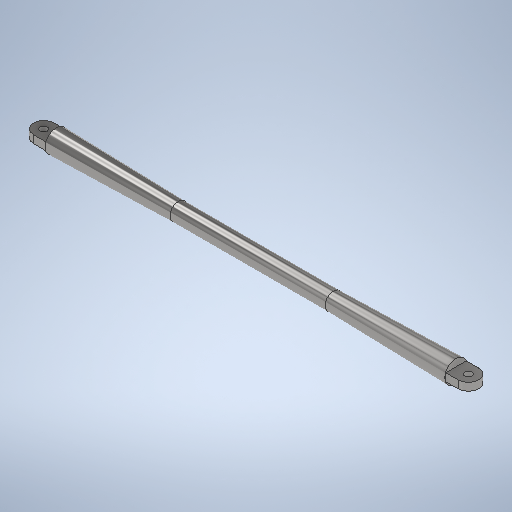
# Autodesk Inventor part: Arjun_SteeringRod
Saved by Autodesk Inventor 2025 (Build 290162000, 162)
## iProperties
Created: 2024-11-03
Part Number: Arjun_SteeringRod
Material: Generic
Document SubType Name: Modeling
Designer: pathl
Density: 1 g/cm^3
Appearance: Default
Author: pathl
Autodesk Inventor part; units mm, degrees
ref_plane "YZ Plane" through (0, 0, 0) normal (1, 0, 0) x (0, 1, 0)
ref_plane "XZ Plane" through (0, 0, 0) normal (0, 1, 0) x (-1, 0, 0)
sketch "Sketch1" plane through (0, 0, 0) normal (0, 0, 1) x (1, 0, 0)
  line L0 (0, 0) -> (575, 0)
  line L1 (575, 0) -> (575, 30)
  line L2 (575, 30) -> (200, 22)
  line L3 (200, 22) -> (0, 22)
  line L4 (0, 22) -> (0, 0)
  dimension "d0" = 575
  dimension "d1" = 30
  dimension "d2" = 22
  dimension "d3" = 200
  constraints: 10 end point, 2 perpendicular, 1 horizontal, 1 parallel
  measures "d0" distance of L0.start L0.end
  measures "d1" distance of L0.end L1.end
  measures "d2" distance of L3.end L0.start
  measures "d3" distance of L2.end L3.end
revolve "Revolution1" add sketch "Sketch1" angle 360 about axis through (0, 0, 0) along (1, 0, 0)
ref_plane "Work Plane1" through (0, 0, 30) normal (0, 0, 1) x (1, 0, 0)
sketch "Sketch2" plane through (0, 0, 30) normal (0, 0, 1) x (1, 0, 0)
  line L0 (515, 39.8306) -> (599.6476, 39.8306)
  line L1 (599.6476, 39.8306) -> (599.6476, 10)
  line L2 (599.6476, 10) -> (515, 10)
  line L3 (515, 10) -> (515, 39.8306)
  line L4 (509.4984, 0) -> (515, 0)
  line L5 (575, -30) -> (575, 30) projected
  line L6 (512.2492, 0) -> (602.6525, 0)
  line L7 (515, -39.8306) -> (599.6476, -39.8306)
  line L8 (599.6476, -39.8306) -> (599.6476, -10)
  line L9 (599.6476, -10) -> (515, -10)
  line L10 (515, -10) -> (515, -39.8306)
  point P0 (0, 0)
  dimension "d6" = 60
  dimension "d7" = 10
  constraints: 20 end point, 4 symmetric about line, 3 horizontal, 2 parallel, 1 midpoint, 1 perpendicular, 1 point on line
  measures "d6" distance between parallel lines of L5 L3
  measures "d7" distance between parallel lines of L6 L2
extrude "Extrusion1" cut sketch "Sketch2" along normal through all both and the other way through all
sketch "Sketch3" plane through (575, 10, 28.2843) normal (0, 1, 0) x (1, 0, 0)
  line L0 (-60, 55.2071) -> (-60, 1.3614) projected
  line L1 (-60, 55.2071) -> (-28.0755, 55.2071)
  line L2 (-28.0755, 2.2843) -> (-60, 2.2843)
  line L3 (-60, 55.2071) -> (-60, 2.2843)
  arc A0 (-28.0755, 2.2843) -> (-28.0755, 55.2071) centre (-28.0755, 28.7457) ccw
  line L4 (-60, 65.181) -> (5.1582, 65.181)
  line L5 (5.1582, 65.181) -> (5.1582, -12.094)
  line L6 (5.1582, -12.094) -> (-60, -12.094)
  line L7 (-60, -12.094) -> (-60, 65.181)
  point P0 (-575, 28.2843)
  point P1 (-60, 1.3614)
  constraints: 14 end point, 3 horizontal, 2 perpendicular, 2 point on circle, 1 centre point
extrude "Extrusion2" cut sketch "Sketch3" along normal through all both and the other way through all contours L7 L4 L5 L6 L0 L2 A0 L1
sketch "Sketch4" plane through (515, 10, -26.9228) normal (0, 1, 0) x (1, 0, 0)
  circle A0 centre (31.9245, -26.9228) radius 9.5
  point P0 (-515, -26.9228)
  dimension "d12" = 19
  constraints: 1 centre point
  measures "d12" diameter of A0
extrude "Extrusion3" cut sketch "Sketch4" against normal through all
mirror "Mirror1" about plane through (0, 0, 0) normal (1, 0, 0) of "Revolution1", "Extrusion2", "Extrusion3", "Extrusion1"
body "Solid1"
